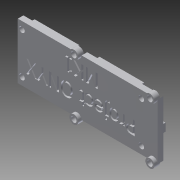
# Autodesk Inventor part: RearCarriageCarrierPlate
Saved by Autodesk Inventor 2015 (Build 190159000, 159)
## iProperties
Created: 2015-05-13
Part Number: RearCarriageCarrierPlate
Material: ABS Plastic
Document SubType Name: Modeling
Designer: Quinn
Density: 1.06 g/cm^3
Appearance: Smooth - White
Author: Quinn
Autodesk Inventor part; units mm, degrees
ref_plane "YZ Plane" through (0, 0, 0) normal (1, 0, 0) x (0, 1, 0)
ref_plane "XZ Plane" through (0, 0, 0) normal (0, 1, 0) x (-1, 0, 0)
ref_plane "XY Plane" through (0, 0, 0) normal (0, 0, 1) x (1, 0, 0)
sketch "Sketch1" plane through (0, 0, 0) normal (0, 1, 0) x (-1, 0, 0)
  line L0 (57, 25) -> (-57, 25)
  line L1 (-57, 25) -> (-57, -25)
  line L2 (-57, -25) -> (57, -25)
  line L3 (57, -25) -> (57, 25)
  point P0 (0, 0)
  point P1 (0, -25)
  point P2 (-57, 0)
  dimension "d0" = 114
  dimension "d1" = 50
  constraints: 8 end point, 2 midpoint, 2 parallel, 1 horizontal, 1 horizontal alignment, 1 perpendicular, 1 vertical alignment
  measures "d0" distance of L2.end L1.end
  measures "d1" distance of L1.end L0.end
extrude "Extrusion1" add sketch "Sketch1" along normal blind 5
sketch "Sketch2" plane through (0, 5, 0) normal (0, 1, 0) x (1, 0, 0)
  line L0 (-57, -25) -> (57, -25) projected
  line L1 (57, -25) -> (57, 25) projected
  line L2 (57, 25) -> (-57, 25) projected
  line L3 (-57, 25) -> (-57, -25) projected
  line L4 (57, -25) -> (49, -25)
  line L5 (49, -25) -> (49, 25)
  line L6 (49, 25) -> (57, 25)
  line L7 (57, 25) -> (57, -25)
  line L8 (49, -25) -> (9, -25)
  line L9 (9, -25) -> (9, 25)
  line L10 (9, 25) -> (49, 25)
  line L11 (49, 25) -> (49, -25)
  line L12 (-57, -25) -> (-49, -25)
  line L13 (-49, -25) -> (-49, 25)
  line L14 (-49, 25) -> (-57, 25)
  line L15 (-57, 25) -> (-57, -25)
  line L16 (-49, -25) -> (-9, -25)
  line L17 (-9, -25) -> (-9, 25)
  line L18 (-9, 25) -> (-49, 25)
  line L19 (-49, 25) -> (-49, -25)
  point P0 (0, 0)
  dimension "d4" = 8
  dimension "d5" = 40
  dimension "d6" = 8
  dimension "d7" = 40
  constraints: 32 end point, 8 parallel, 4 horizontal, 4 perpendicular, 4 point on line
  measures "d4" distance of L5.end L6.end
  measures "d5" distance of L9.end L10.end
  measures "d6" distance of L14.end L13.end
  measures "d7" distance of L18.end L17.end
extrude "Extrusion2" add sketch "Sketch2" along normal blind 2 contours L13 L2 L17 L0 | L9 L2 L5 L0
sketch "Sketch3" plane through (0, 0, 0) normal (0, -1, 0) x (1, 0, 0)
  line L0 (-57, 25) -> (57, 25) projected
  line L1 (-57, -25) -> (-57, 25) projected
  line L2 (57, -25) -> (-57, -25) projected
  line L3 (57, 25) -> (57, -25) projected
  line L4 (-57, 0) -> (57, 0)
  line L5 (-57, -25) -> (-57, -12.5)
  point P0 (0, 0)
  constraints: 4 end point, 2 midpoint, 1 point on line
sketch "Sketch4" plane through (0, 5, 0) normal (0, 1, 0) x (1, 0, 0)
  line L0 (9, -25) -> (9, 25) projected
  line L1 (9, 25) -> (-9, 25) projected
  line L2 (-9, 25) -> (-9, -25) projected
  line L3 (-9, -25) -> (9, -25) projected
  line L4 (49, 25) -> (49, -25) projected
  line L5 (49, -25) -> (57, -25) projected
  line L6 (57, -25) -> (57, 25) projected
  line L7 (57, 25) -> (49, 25) projected
  line L8 (-49, -25) -> (-49, 25) projected
  line L9 (-49, 25) -> (-57, 25) projected
  line L10 (-57, 25) -> (-57, -25) projected
  line L11 (-57, -25) -> (-49, -25) projected
  line L12 (-57, 3.5) -> (-49, 3.5)
  line L13 (-49, 3.5) -> (-49, -3.5)
  line L14 (-49, -3.5) -> (-57, -3.5)
  line L15 (-57, -3.5) -> (-57, 3.5)
  line L16 (-57, 3.5) -> (-49, -3.5) construction
  line L17 (-49, 3.5) -> (-57, -3.5) construction
  line L18 (-9, 3.5) -> (9, 3.5)
  line L19 (9, 3.5) -> (9, -3.5)
  line L20 (9, -3.5) -> (-9, -3.5)
  line L21 (-9, -3.5) -> (-9, 3.5)
  line L22 (-9, 3.5) -> (9, -3.5) construction
  line L23 (9, 3.5) -> (-9, -3.5) construction
  line L24 (49, 3.5) -> (57, 3.5)
  line L25 (57, 3.5) -> (57, -3.5)
  line L26 (57, -3.5) -> (49, -3.5)
  line L27 (49, -3.5) -> (49, 3.5)
  line L28 (49, 3.5) -> (57, -3.5) construction
  line L29 (57, 3.5) -> (49, -3.5) construction
  point P0 (0, 0)
  point P1 (-53, 0)
  point P2 (53, 0)
  dimension "d11" = 7
  constraints: 36 end point, 6 midpoint, 6 parallel, 5 point on line, 3 horizontal, 3 perpendicular
  measures "d11" distance of L12.end L13.end
extrude "Extrusion3" add sketch "Sketch4" along normal blind 2 contours L20 L2 L18 L0 | L24 L6 L26 L4 | L14 L10 L12 L8
sketch "Sketch5" plane through (0, 0, 0) normal (0, -1, 0) x (1, 0, 0)
  line L0 (-57, 25) -> (57, 25) projected
  line L1 (-57, -25) -> (-57, 25) projected
  line L2 (57, -25) -> (-57, -25) projected
  line L3 (57, 25) -> (57, -25) projected
  line L4 (-9, -25) -> (-49, -25) projected
  line L5 (-49, -25) -> (-49, -3.5) projected
  line L6 (-49, -3.5) -> (-57, -3.5) projected
  line L7 (-57, -3.5) -> (-57, 3.5) projected
  line L8 (-57, 3.5) -> (-49, 3.5) projected
  line L9 (-49, 3.5) -> (-49, 25) projected
  line L10 (-49, 25) -> (-9, 25) projected
  line L11 (-9, 25) -> (-9, 3.5) projected
  line L12 (-9, 3.5) -> (9, 3.5) projected
  line L13 (9, 3.5) -> (9, 25) projected
  line L14 (9, 25) -> (49, 25) projected
  line L15 (49, 25) -> (49, 3.5) projected
  line L16 (49, 3.5) -> (57, 3.5) projected
  line L17 (57, 3.5) -> (57, -3.5) projected
  line L18 (57, -3.5) -> (49, -3.5) projected
  line L19 (49, -3.5) -> (49, -25) projected
  line L20 (49, -25) -> (9, -25) projected
  line L21 (9, -25) -> (9, -3.5) projected
  line L22 (9, -3.5) -> (-9, -3.5) projected
  line L23 (-9, -3.5) -> (-9, -25) projected
  line L24 (-9, 25) -> (-4, 25)
  line L25 (-4, 25) -> (-4, -25)
  circle A0 centre (-4, -25) radius 4
  circle A1 centre (-4, 25) radius 4
  circle A2 centre (-4, 25) radius 2.5
  circle A3 centre (-4, -25) radius 2.5
  line L26 (-4, -25) -> (64, -25)
  line L27 (64, -25) -> (64, 25)
  circle A4 centre (64, -25) radius 4
  circle A5 centre (64, 25) radius 4
  circle A6 centre (64, -25) radius 2.5
  circle A7 centre (64, 25) radius 2.5
  point P0 (0, 0)
  dimension "d14" = 5
  dimension "d15" = 8
  dimension "d16" = 8
  dimension "d17" = 5
  dimension "d18" = 5
  dimension "d19" = 68
  dimension "d20" = 8
  dimension "d21" = 8
  dimension "d22" = 5
  dimension "d23" = 5
  constraints: 8 centre point, 8 coincident, 8 end point, 3 point on line, 2 perpendicular
  measures "d14" distance of L10.end L24.end
  measures "d15" diameter of A0
  measures "d16" diameter of A1
  measures "d17" diameter of A2
  measures "d18" diameter of A3
  measures "d19" distance of L26.start L26.end
  measures "d20" diameter of A4
  measures "d21" diameter of A5
  measures "d22" diameter of A6
  measures "d23" diameter of A7
move faces "Move1" translate (11, 0, 0) faces at (57, 1.6667, 1.1667)
extrude "Extrusion4" cut sketch "Sketch5" against normal blind 5 contours A2 L0 | L0 L25 A2 | L0 A2 L25 | A3 L2 L25 | L25 L2 A3 | L2 A3 | A6 L27 L26 | L26 L27 A6 | A7
extrude "Extrusion5" add sketch "Sketch5" against normal blind 5 contours A1 L0 A2 | L0 A2 L25 A1 | A1 L25 A2 L0 | A0 L2 A3 L25 | L25 A3 L2 A0 | L2 A3 A0 | A4 L27 A6 L26 | L26 A6 L27 A4 | A5
extrude "Extrusion6" add sketch "Sketch5" along normal blind 3 contours A1 L0 A2 | L0 A2 L25 A1 | A1 L25 A2 L0 | A0 L2 A3 L25 | L25 A3 L2 A0 | L2 A3 A0 | A4 L27 A6 L26 | L26 A6 L27 A4 | A5
sketch "Sketch6" plane through (0, 0, 0) normal (0, -1, 0) x (1, 0, 0)
  arc A0 (-8, 25) -> (0, 25) centre (-4, 25) ccw projected
  line L0 (-57, 25) -> (-8, 25) projected
  line L1 (-57, -25) -> (-57, 25) projected
  line L2 (-8, -25) -> (-57, -25) projected
  arc A1 (0, -25) -> (-8, -25) centre (-4, -25) ccw projected
  line L3 (60, -25) -> (0, -25) projected
  arc A2 (68, -25) -> (60, -25) centre (64, -25) ccw projected
  line L4 (68, 25) -> (68, -25) projected
  arc A3 (60, 25) -> (68, 25) centre (64, 25) ccw projected
  line L5 (0, 25) -> (60, 25) projected
  line L6 (185.6734, -14.1018) -> (-186.4568, -14.1018) construction
  line L7 (-186.4568, -14.1018) -> (-186.4568, 105.3716) construction
  line L8 (-186.4568, 105.3716) -> (185.6734, 105.3716) construction
  line L9 (185.6734, 105.3716) -> (185.6734, -14.1018) construction
  spline S0 degree 2 poles (39.8019, -10.2039) (39.8019, -9.4204) (40.3601, -8.0101) (40.8596, -7.5204) knots 0 0 0 1 2 2 2
  spline S1 degree 2 poles (40.8596, -7.5204) (41.4864, -6.9034) (43.1807, -6.2668) (44.4735, -6.2668) knots 0 0 0 1 2 2 2
  line L10 (44.4735, -6.2668) -> (45.8348, -6.2668)
  line L11 (45.8348, -6.2668) -> (45.8348, -1.7616)
  line L12 (45.8348, -1.7616) -> (47.441, -1.7616)
  line L13 (47.441, -1.7616) -> (47.441, -13.8471)
  line L14 (47.441, -13.8471) -> (44.4049, -13.8471)
  spline S2 degree 2 poles (44.4049, -13.8471) (43.3276, -13.8471) (41.8194, -13.4946) (41.2416, -13.093) knots 0 0 0 1 2 2 2
  spline S3 degree 2 poles (41.2416, -13.093) (40.5658, -12.6327) (39.8019, -11.2126) (39.8019, -10.2039) knots 0 0 0 1 2 2 2
  spline S4 degree 2 poles (41.4766, -10.1549) (41.4766, -10.7817) (41.9075, -11.7023) (42.3483, -11.9961) knots 0 0 0 1 2 2 2
  spline S5 degree 2 poles (42.3483, -11.9961) (42.7302, -12.2508) (43.7488, -12.4564) (44.5029, -12.4564) knots 0 0 0 1 2 2 2
  line L15 (44.5029, -12.4564) -> (45.8348, -12.4564)
  line L16 (45.8348, -12.4564) -> (45.8348, -7.6379)
  line L17 (45.8348, -7.6379) -> (44.7379, -7.6379)
  spline S6 degree 2 poles (44.7379, -7.6379) (43.7586, -7.6379) (42.5539, -7.9513) (42.1622, -8.3626) knots 0 0 0 1 2 2 2
  spline S7 degree 2 poles (42.1622, -8.3626) (41.7998, -8.725) (41.4766, -9.5771) (41.4766, -10.1549) knots 0 0 0 1 2 2 2
  line L18 (33.5828, -9.1951) -> (33.6612, -9.1951)
  spline S8 degree 2 poles (33.6612, -9.1951) (33.8375, -9.2441) (34.2194, -9.2637) (34.4839, -9.2637) knots 0 0 0 1 2 2 2
  spline S9 degree 2 poles (34.4839, -9.2637) (35.1009, -9.2637) (36.3153, -8.725) (36.8637, -8.1961) knots 0 0 0 1 2 2 2
  line L19 (36.8637, -8.1961) -> (36.8637, -1.7616)
  line L20 (36.8637, -1.7616) -> (38.3916, -1.7616)
  line L21 (38.3916, -1.7616) -> (38.3916, -10.8307)
  line L22 (38.3916, -10.8307) -> (36.8637, -10.8307)
  line L23 (36.8637, -10.8307) -> (36.8637, -9.4791)
  spline S10 degree 2 poles (36.8637, -9.4791) (36.0313, -10.2234) (34.7875, -10.8307) (34.1998, -10.8307) knots 0 0 0 1 2 2 2
  spline S11 degree 2 poles (34.1998, -10.8307) (33.9648, -10.8307) (33.7297, -10.8111) (33.5828, -10.7817) knots 0 0 0 1 2 2 2
  line L24 (33.5828, -10.7817) -> (33.5828, -9.1951)
  spline S12 degree 2 poles (24.9447, -6.2961) (24.9447, -4.0044) (27.1483, -1.507) (28.9896, -1.507) knots 0 0 0 1 2 2 2
  spline S13 degree 2 poles (28.9896, -1.507) (30.8798, -1.507) (33.0442, -4.0828) (33.0442, -6.2961) knots 0 0 0 1 2 2 2
  spline S14 degree 2 poles (33.0442, -6.2961) (33.0442, -8.5683) (30.8112, -11.0853) (28.9896, -11.0853) knots 0 0 0 1 2 2 2
  spline S15 degree 2 poles (28.9896, -11.0853) (27.1483, -11.0853) (24.9447, -8.5781) (24.9447, -6.2961) knots 0 0 0 1 2 2 2
  spline S16 degree 2 poles (26.5215, -6.2961) (26.5215, -8.059) (27.8045, -9.7729) (28.9896, -9.7729) knots 0 0 0 1 2 2 2
  spline S17 degree 2 poles (28.9896, -9.7729) (30.1746, -9.7729) (31.4674, -8.059) (31.4674, -6.2961) knots 0 0 0 1 2 2 2
  spline S18 degree 2 poles (31.4674, -6.2961) (31.4674, -4.5822) (30.1746, -2.8194) (28.9896, -2.8194) knots 0 0 0 1 2 2 2
  spline S19 degree 2 poles (28.9896, -2.8194) (27.8143, -2.8194) (26.5215, -4.5529) (26.5215, -6.2961) knots 0 0 0 1 2 2 2
  spline S20 degree 2 poles (20.9097, -1.507) (20.9097, 0.0404) (22.5747, 1.6662) (24.0339, 1.6662) knots 0 0 0 1 2 2 2
  spline S21 degree 2 poles (24.0339, 1.6662) (24.2886, 1.6662) (24.9154, 1.6172) (25.219, 1.5682) knots 0 0 0 1 2 2 2
  line L25 (25.219, 1.5682) -> (25.219, 0.1971)
  line L26 (25.219, 0.1971) -> (25.1308, 0.1971)
  spline S22 degree 2 poles (25.1308, 0.1971) (24.9545, 0.2363) (24.5236, 0.3146) (24.3277, 0.3146) knots 0 0 0 1 2 2 2
  spline S23 degree 2 poles (24.3277, 0.3146) (23.7205, 0.3146) (22.9272, 0.011) (22.7411, -0.3122) knots 0 0 0 1 2 2 2
  spline S24 degree 2 poles (22.7411, -0.3122) (22.5551, -0.606) (22.4375, -1.4972) (22.4375, -2.1338) knots 0 0 0 1 2 2 2
  line L27 (22.4375, -2.1338) -> (22.4375, -9.5673)
  line L28 (22.4375, -9.5673) -> (24.0731, -9.5673)
  line L29 (24.0731, -9.5673) -> (24.0731, -10.8307)
  line L30 (24.0731, -10.8307) -> (20.9097, -10.8307)
  line L31 (20.9097, -10.8307) -> (20.9097, -1.507)
  line L32 (20.8999, -12.3389) -> (22.6334, -12.3389)
  line L33 (22.6334, -12.3389) -> (22.6334, -13.9255)
  line L34 (22.6334, -13.9255) -> (20.8999, -13.9255)
  line L35 (20.8999, -13.9255) -> (20.8999, -12.3389)
  spline S25 degree 2 poles (14.7592, -1.556) (16.9334, -1.556) (19.3231, -3.9946) (19.3231, -6.2472) knots 0 0 0 1 2 2 2
  spline S26 degree 2 poles (19.3231, -6.2472) (19.3231, -8.4606) (17.002, -11.0853) (15.1314, -11.0853) knots 0 0 0 1 2 2 2
  spline S27 degree 2 poles (15.1314, -11.0853) (14.2891, -11.0853) (12.9866, -10.5956) (12.5067, -10.0765) knots 0 0 0 1 2 2 2
  spline S28 degree 2 poles (12.5067, -10.0765) (12.017, -9.5575) (11.4979, -8.059) (11.4979, -6.9719) knots 0 0 0 1 2 2 2
  line L36 (11.4979, -6.9719) -> (11.4979, -6.1394)
  line L37 (11.4979, -6.1394) -> (17.7757, -6.1394)
  spline S29 degree 2 poles (17.7757, -6.1394) (17.7757, -4.5627) (16.1891, -2.8879) (14.7788, -2.8879) knots 0 0 0 1 2 2 2
  spline S30 degree 2 poles (14.7788, -2.8879) (14.2793, -2.8879) (13.3098, -3.1132) (12.918, -3.2895) knots 0 0 0 1 2 2 2
  spline S31 degree 2 poles (12.918, -3.2895) (12.5067, -3.4853) (11.9386, -3.8281) (11.7525, -3.9848) knots 0 0 0 1 2 2 2
  line L38 (11.7525, -3.9848) -> (11.6644, -3.9848)
  line L39 (11.6644, -3.9848) -> (11.6644, -2.3199)
  spline S32 degree 2 poles (11.6644, -2.3199) (11.9288, -2.2122) (12.7319, -1.8988) (13.0453, -1.8106) knots 0 0 0 1 2 2 2
  spline S33 degree 2 poles (13.0453, -1.8106) (13.486, -1.6833) (14.2108, -1.556) (14.7592, -1.556) knots 0 0 0 1 2 2 2
  spline S34 degree 2 poles (12.9866, -7.3049) (13.0061, -7.9219) (13.2608, -8.8229) (13.5056, -9.1265) knots 0 0 0 1 2 2 2
  spline S35 degree 2 poles (13.5056, -9.1265) (13.7701, -9.4693) (14.6025, -9.8317) (15.2195, -9.8317) knots 0 0 0 1 2 2 2
  spline S36 degree 2 poles (15.2195, -9.8317) (15.8268, -9.8317) (16.6788, -9.4693) (17.0314, -9.1168) knots 0 0 0 1 2 2 2
  spline S37 degree 2 poles (17.0314, -9.1168) (17.3742, -8.7544) (17.7267, -7.8827) (17.7757, -7.3049) knots 0 0 0 1 2 2 2
  line L40 (17.7757, -7.3049) -> (12.9866, -7.3049)
  spline S38 degree 2 poles (6.3464, -1.556) (7.2866, -1.556) (8.8438, -2.1338) (9.402, -2.7214) knots 0 0 0 1 2 2 2
  spline S39 degree 2 poles (9.402, -2.7214) (9.9603, -3.2993) (10.5773, -5.0817) (10.5773, -6.2766) knots 0 0 0 1 2 2 2
  spline S40 degree 2 poles (10.5773, -6.2766) (10.5773, -7.4714) (9.9407, -9.2147) (9.402, -9.8023) knots 0 0 0 1 2 2 2
  spline S41 degree 2 poles (9.402, -9.8023) (8.8634, -10.3997) (7.267, -11.0363) (6.3464, -11.0363) knots 0 0 0 1 2 2 2
  spline S42 degree 2 poles (6.3464, -11.0363) (5.6021, -11.0363) (4.2114, -10.6152) (3.6727, -10.341) knots 0 0 0 1 2 2 2
  line L41 (3.6727, -10.341) -> (3.6727, -8.6271)
  line L42 (3.6727, -8.6271) -> (3.7608, -8.6271)
  spline S43 degree 2 poles (3.7608, -8.6271) (3.9273, -8.7642) (4.4366, -9.1168) (4.799, -9.3028) knots 0 0 0 1 2 2 2
  spline S44 degree 2 poles (4.799, -9.3028) (5.1222, -9.4595) (5.984, -9.7044) (6.3758, -9.7044) knots 0 0 0 1 2 2 2
  spline S45 degree 2 poles (6.3758, -9.7044) (7.5608, -9.7044) (9.0005, -7.9121) (9.0005, -6.2766) knots 0 0 0 1 2 2 2
  spline S46 degree 2 poles (9.0005, -6.2766) (9.0005, -4.6802) (7.6098, -2.8879) (6.3758, -2.8879) knots 0 0 0 1 2 2 2
  spline S47 degree 2 poles (6.3758, -2.8879) (5.6314, -2.8879) (4.2799, -3.5049) (3.7608, -3.9848) knots 0 0 0 1 2 2 2
  line L43 (3.7608, -3.9848) -> (3.6727, -3.9848)
  line L44 (3.6727, -3.9848) -> (3.6727, -2.2709)
  spline S48 degree 2 poles (3.6727, -2.2709) (3.898, -2.1632) (4.5835, -1.8596) (4.8577, -1.791) knots 0 0 0 1 2 2 2
  spline S49 degree 2 poles (4.8577, -1.791) (5.2495, -1.6735) (5.8665, -1.556) (6.3464, -1.556) knots 0 0 0 1 2 2 2
  spline S50 degree 2 poles (-0.4603, -1.5854) (0.7835, -1.5854) (2.184, -3.0054) (2.184, -4.5431) knots 0 0 0 1 2 2 2
  line L45 (2.184, -4.5431) -> (2.184, -9.5673)
  line L46 (2.184, -9.5673) -> (3.2124, -9.5673)
  line L47 (3.2124, -9.5673) -> (3.2124, -10.8307)
  line L48 (3.2124, -10.8307) -> (2.184, -10.8307)
  line L49 (2.184, -10.8307) -> (2.184, -13.4358)
  line L50 (2.184, -13.4358) -> (0.6562, -13.4358)
  line L51 (0.6562, -13.4358) -> (0.6562, -10.8307)
  line L52 (0.6562, -10.8307) -> (-2.1546, -10.8307)
  line L53 (-2.1546, -10.8307) -> (-2.1546, -9.5673)
  line L54 (-2.1546, -9.5673) -> (0.6562, -9.5673)
  line L55 (0.6562, -9.5673) -> (0.6562, -5.2482)
  spline S51 degree 2 poles (0.6562, -5.2482) (0.6562, -4.5627) (0.6072, -3.8085) (0.4408, -3.4853) knots 0 0 0 1 2 2 2
  spline S52 degree 2 poles (0.4408, -3.4853) (0.3036, -3.2013) (-0.3134, -2.9173) (-0.8422, -2.9173) knots 0 0 0 1 2 2 2
  spline S53 degree 2 poles (-0.8422, -2.9173) (-1.2144, -2.9173) (-1.9097, -3.1426) (-2.0664, -3.2111) knots 0 0 0 1 2 2 2
  line L56 (-2.0664, -3.2111) -> (-2.1546, -3.2111)
  line L57 (-2.1546, -3.2111) -> (-2.1546, -1.84)
  spline S54 degree 2 poles (-2.1546, -1.84) (-1.7237, -1.7225) (-0.8422, -1.5854) (-0.4603, -1.5854) knots 0 0 0 1 2 2 2
  spline S55 degree 2 poles (-17.139, -12.4662) (-17.8246, -11.6631) (-18.5885, -9.3126) (-18.5885, -7.8044) knots 0 0 0 1 2 2 2
  spline S56 degree 2 poles (-18.5885, -7.8044) (-18.5885, -6.3353) (-17.8442, -3.9554) (-17.139, -3.1524) knots 0 0 0 1 2 2 2
  spline S57 degree 2 poles (-17.139, -3.1524) (-16.3947, -2.3101) (-14.4262, -1.507) (-13.2411, -1.507) knots 0 0 0 1 2 2 2
  spline S58 degree 2 poles (-13.2411, -1.507) (-12.0169, -1.507) (-10.0582, -2.3395) (-9.3432, -3.1524) knots 0 0 0 1 2 2 2
  spline S59 degree 2 poles (-9.3432, -3.1524) (-8.6479, -3.9554) (-7.9035, -6.3157) (-7.9035, -7.8044) knots 0 0 0 1 2 2 2
  spline S60 degree 2 poles (-7.9035, -7.8044) (-7.9035, -9.3224) (-8.6576, -11.6337) (-9.353, -12.4662) knots 0 0 0 1 2 2 2
  spline S61 degree 2 poles (-9.353, -12.4662) (-10.0582, -13.2693) (-12.0267, -14.1018) (-13.2411, -14.1018) knots 0 0 0 1 2 2 2
  spline S62 degree 2 poles (-13.2411, -14.1018) (-14.4751, -14.1018) (-16.4535, -13.2399) (-17.139, -12.4662) knots 0 0 0 1 2 2 2
  spline S63 degree 2 poles (-16.9138, -7.8044) (-16.9138, -8.9992) (-16.3947, -10.8502) (-15.9246, -11.4575) knots 0 0 0 1 2 2 2
  spline S64 degree 2 poles (-15.9246, -11.4575) (-15.4447, -12.0843) (-14.0932, -12.7111) (-13.2509, -12.7111) knots 0 0 0 1 2 2 2
  spline S65 degree 2 poles (-13.2509, -12.7111) (-12.3793, -12.7111) (-11.0669, -12.1038) (-10.5674, -11.4575) knots 0 0 0 1 2 2 2
  spline S66 degree 2 poles (-10.5674, -11.4575) (-10.0875, -10.8405) (-9.5783, -8.9796) (-9.5783, -7.8044) knots 0 0 0 1 2 2 2
  spline S67 degree 2 poles (-9.5783, -7.8044) (-9.5783, -5.4245) (-11.5762, -2.8977) (-13.2509, -2.8977) knots 0 0 0 1 2 2 2
  spline S68 degree 2 poles (-13.2509, -2.8977) (-14.9257, -2.8977) (-16.9138, -5.4245) (-16.9138, -7.8044) knots 0 0 0 1 2 2 2
  line L58 (-28.9993, -1.7616) -> (-27.1972, -1.7616)
  line L59 (-27.1972, -1.7616) -> (-21.8498, -12.1822)
  line L60 (-21.8498, -12.1822) -> (-21.8498, -1.7616)
  line L61 (-21.8498, -1.7616) -> (-20.3514, -1.7616)
  line L62 (-20.3514, -1.7616) -> (-20.3514, -13.8471)
  line L63 (-20.3514, -13.8471) -> (-22.6333, -13.8471)
  line L64 (-22.6333, -13.8471) -> (-27.5008, -4.2786)
  line L65 (-27.5008, -4.2786) -> (-27.5008, -13.8471)
  line L66 (-27.5008, -13.8471) -> (-28.9993, -13.8471)
  line L67 (-28.9993, -13.8471) -> (-28.9993, -1.7616)
  line L68 (-39.9095, -13.8471) -> (-35.8255, -7.109)
  line L69 (-35.8255, -7.109) -> (-35.8255, -1.7616)
  line L70 (-35.8255, -1.7616) -> (-34.2194, -1.7616)
  line L71 (-34.2194, -1.7616) -> (-34.2194, -6.9425)
  line L72 (-34.2194, -6.9425) -> (-30.1354, -13.8471)
  line L73 (-30.1354, -13.8471) -> (-31.9178, -13.8471)
  line L74 (-31.9178, -13.8471) -> (-35.0322, -8.5291)
  line L75 (-35.0322, -8.5291) -> (-38.2054, -13.8471)
  line L76 (-38.2054, -13.8471) -> (-39.9095, -13.8471)
  line L77 (-49.3801, -1.7616) -> (-47.5389, -1.7616)
  line L78 (-47.5389, -1.7616) -> (-44.6007, -6.5802)
  line L79 (-44.6007, -6.5802) -> (-41.6039, -1.7616)
  line L80 (-41.6039, -1.7616) -> (-39.8704, -1.7616)
  line L81 (-39.8704, -1.7616) -> (-43.7193, -7.8142)
  line L82 (-43.7193, -7.8142) -> (-39.9879, -13.8471)
  line L83 (-39.9879, -13.8471) -> (-41.8291, -13.8471)
  line L84 (-41.8291, -13.8471) -> (-44.7085, -9.1168)
  line L85 (-44.7085, -9.1168) -> (-47.6466, -13.8471)
  line L86 (-47.6466, -13.8471) -> (-49.3801, -13.8471)
  line L87 (-49.3801, -13.8471) -> (-45.5997, -7.8925)
  line L88 (-45.5997, -7.8925) -> (-49.3801, -1.7616)
  line L89 (3.849, 18.1368) -> (5.4552, 18.1368)
  line L90 (5.4552, 18.1368) -> (5.4552, 7.7261)
  line L91 (5.4552, 7.7261) -> (8.6087, 14.8069)
  line L92 (8.6087, 14.8069) -> (9.5881, 14.8069)
  line L93 (9.5881, 14.8069) -> (12.7123, 7.7261)
  line L94 (12.7123, 7.7261) -> (12.7123, 18.1368)
  line L95 (12.7123, 18.1368) -> (14.2108, 18.1368)
  line L96 (14.2108, 18.1368) -> (14.2108, 6.0513)
  line L97 (14.2108, 6.0513) -> (12.017, 6.0513)
  line L98 (12.017, 6.0513) -> (9.0005, 12.7796)
  line L99 (9.0005, 12.7796) -> (6.082, 6.0513)
  line L100 (6.082, 6.0513) -> (3.849, 6.0513)
  line L101 (3.849, 6.0513) -> (3.849, 18.1368)
  line L102 (-7.4138, 18.1368) -> (-5.3278, 18.1368)
  line L103 (-5.3278, 18.1368) -> (-0.9108, 12.5152)
  line L104 (-0.9108, 12.5152) -> (-0.2056, 13.3085)
  line L105 (-0.2056, 13.3085) -> (-0.2056, 18.1368)
  line L106 (-0.2056, 18.1368) -> (1.4005, 18.1368)
  line L107 (1.4005, 18.1368) -> (1.4005, 6.0513)
  line L108 (1.4005, 6.0513) -> (-0.2056, 6.0513)
  line L109 (-0.2056, 6.0513) -> (-0.2056, 11.6044)
  line L110 (-0.2056, 11.6044) -> (-5.1613, 6.0513)
  line L111 (-5.1613, 6.0513) -> (-7.12, 6.0513)
  line L112 (-7.12, 6.0513) -> (-2.1154, 11.4477)
  line L113 (-2.1154, 11.4477) -> (-7.4138, 18.1368)
  line L114 (-14.8767, 18.1368) -> (-8.9808, 18.1368)
  line L115 (-8.9808, 18.1368) -> (-8.9808, 16.9028)
  line L116 (-8.9808, 16.9028) -> (-11.1746, 16.9028)
  line L117 (-11.1746, 16.9028) -> (-11.1746, 8.8034)
  line L118 (-11.1746, 8.8034) -> (-8.9808, 8.8034)
  line L119 (-8.9808, 8.8034) -> (-8.9808, 7.6967)
  spline S69 degree 2 poles (-8.9808, 7.6967) (-10.2247, 7.6967) (-11.3999, 6.9915) (-11.4783, 6.0121) knots 0 0 0 1 2 2 2
  line L120 (-11.4783, 6.0121) -> (-12.7319, 6.0121)
  line L121 (-12.7319, 6.0121) -> (-12.7319, 16.9028)
  line L122 (-12.7319, 16.9028) -> (-14.8767, 16.9028)
  line L123 (-14.8767, 16.9028) -> (-14.8767, 18.1368)
  point P0 (0, 0)
  constraints: 2 other
emboss "Emboss1" sketch "Sketch6" operation cut depth 2 direction (0, 1, 0) contours S0 S1 L10 L11 L12 L13 L14 S2 S3 | L18 S8 S9 L19 L20 L21 L22 L23 S10 S11 L24 | S12 S13 S14 S15 | S20 S21 L25 L26 S22 S23 S24 L27 L28 L29 L30 L31 | L32 L33 L34 L35 | S25 S26 S27 S28 L36 L37 S29 S30 S31 L38 L39 S32 S33 | S38 S39 S40 S41 S42 L41 L42 S43 S44 S45 S46 S47 L43 L44 S48 S49 | S50 L45 L46 L47 L48 L49 L50 L51 L52 L53 L54 L55 S51 S52 S53 L56 L57 S54 | S55 S56 S57 S58 S59 S60 S61 S62 | L58 L59 L60 L61 L62 L63 L64 L65 L66 L67 | L68 L69 L70 L71 L72 L73 L74 L75 L76 | L77 L78 L79 L80 L81 L82 L83 L84 L85 L86 L87 L88 | L89 L90 L91 L92 L93 L94 L95 L96 L97 L98 L99 L100 L101 | L102 L103 L104 L105 L106 L107 L108 L109 L110 L111 L112 L113 | L114 L115 L116 L117 L118 L119 S69 L120 L121 L122 L123
sketch "Sketch7" plane through (0, 0, 0) normal (0, -1, 0) x (1, 0, 0)
  line L0 (-11.4783, 6.0121) -> (-12.7319, 6.0121) projected
  line L1 (-12.7319, 6.0121) -> (-12.7319, 16.9028) projected
  line L2 (-12.7319, 16.9028) -> (-14.8767, 16.9028) projected
  line L3 (-14.8767, 16.9028) -> (-14.8767, 18.1368) projected
  line L4 (-14.8767, 18.1368) -> (-8.9808, 18.1368) projected
  line L5 (-8.9808, 18.1368) -> (-8.9808, 16.9028) projected
  line L6 (-8.9808, 16.9028) -> (-11.1746, 16.9028) projected
  line L7 (-11.1746, 16.9028) -> (-11.1746, 8.8034) projected
  line L8 (-11.1746, 8.8034) -> (-8.9808, 8.8034) projected
  line L9 (-8.9808, 8.8034) -> (-8.9808, 7.6967) projected
  line L10 (22.4375, -2.1338) -> (22.4375, -9.5673) projected
  line L11 (22.4375, -9.5673) -> (24.0731, -9.5673) projected
  line L12 (24.0731, -9.5673) -> (24.0731, -10.8307) projected
  line L13 (24.0731, -10.8307) -> (20.9097, -10.8307) projected
  line L14 (20.9097, -10.8307) -> (20.9097, -1.507) projected
  line L15 (25.219, 1.5682) -> (25.219, 0.1971) projected
  line L16 (25.219, 0.1971) -> (25.1308, 0.1971) projected
  line L17 (47.441, -13.8471) -> (44.4049, -13.8471) projected
  line L18 (44.4735, -6.2668) -> (45.8348, -6.2668) projected
  line L19 (45.8348, -6.2668) -> (45.8348, -1.7616) projected
  line L20 (45.8348, -1.7616) -> (47.441, -1.7616) projected
  line L21 (47.441, -1.7616) -> (47.441, -13.8471) projected
  line L22 (11.7525, -3.9848) -> (11.6644, -3.9848) projected
  line L23 (11.6644, -3.9848) -> (11.6644, -2.3199) projected
  line L24 (11.4979, -6.9719) -> (11.4979, -6.1394) projected
  line L25 (11.4979, -6.1394) -> (17.7757, -6.1394) projected
  line L26 (36.8637, -10.8307) -> (36.8637, -9.4791) projected
  line L27 (33.5828, -10.7817) -> (33.5828, -9.1951) projected
  line L28 (33.5828, -9.1951) -> (33.6612, -9.1951) projected
  line L29 (36.8637, -8.1961) -> (36.8637, -1.7616) projected
  line L30 (36.8637, -1.7616) -> (38.3916, -1.7616) projected
  line L31 (38.3916, -1.7616) -> (38.3916, -10.8307) projected
  line L32 (38.3916, -10.8307) -> (36.8637, -10.8307) projected
  line L33 (3.7608, -3.9848) -> (3.6727, -3.9848) projected
  line L34 (3.6727, -3.9848) -> (3.6727, -2.2709) projected
  line L35 (3.6727, -10.341) -> (3.6727, -8.6271) projected
  line L36 (3.6727, -8.6271) -> (3.7608, -8.6271) projected
  line L37 (20.8999, -12.3389) -> (22.6334, -12.3389) projected
  line L38 (22.6334, -12.3389) -> (22.6334, -13.9255) projected
  line L39 (22.6334, -13.9255) -> (20.8999, -13.9255) projected
  line L40 (20.8999, -13.9255) -> (20.8999, -12.3389) projected
  line L41 (0.6562, -9.5673) -> (0.6562, -5.2482) projected
  line L42 (-2.0664, -3.2111) -> (-2.1546, -3.2111) projected
  line L43 (-2.1546, -3.2111) -> (-2.1546, -1.84) projected
  line L44 (2.184, -4.5431) -> (2.184, -9.5673) projected
  line L45 (2.184, -9.5673) -> (3.2124, -9.5673) projected
  line L46 (3.2124, -9.5673) -> (3.2124, -10.8307) projected
  line L47 (3.2124, -10.8307) -> (2.184, -10.8307) projected
  line L48 (2.184, -10.8307) -> (2.184, -13.4358) projected
  line L49 (2.184, -13.4358) -> (0.6562, -13.4358) projected
  line L50 (0.6562, -13.4358) -> (0.6562, -10.8307) projected
  line L51 (0.6562, -10.8307) -> (-2.1546, -10.8307) projected
  line L52 (-2.1546, -10.8307) -> (-2.1546, -9.5673) projected
  line L53 (-2.1546, -9.5673) -> (0.6562, -9.5673) projected
  line L54 (-22.6333, -13.8471) -> (-27.5008, -4.2786) projected
  line L55 (-27.5008, -4.2786) -> (-27.5008, -13.8471) projected
  line L56 (-27.5008, -13.8471) -> (-28.9993, -13.8471) projected
  line L57 (-28.9993, -13.8471) -> (-28.9993, -1.7616) projected
  line L58 (-28.9993, -1.7616) -> (-27.1972, -1.7616) projected
  line L59 (-27.1972, -1.7616) -> (-21.8498, -12.1822) projected
  line L60 (-21.8498, -12.1822) -> (-21.8498, -1.7616) projected
  line L61 (-21.8498, -1.7616) -> (-20.3514, -1.7616) projected
  line L62 (-20.3514, -1.7616) -> (-20.3514, -13.8471) projected
  line L63 (-20.3514, -13.8471) -> (-22.6333, -13.8471) projected
  line L64 (-31.9178, -13.8471) -> (-35.0322, -8.5291) projected
  line L65 (-35.0322, -8.5291) -> (-38.2054, -13.8471) projected
  line L66 (-38.2054, -13.8471) -> (-39.9095, -13.8471) projected
  line L67 (-39.9095, -13.8471) -> (-35.8255, -7.109) projected
  line L68 (-35.8255, -7.109) -> (-35.8255, -1.7616) projected
  line L69 (-35.8255, -1.7616) -> (-34.2194, -1.7616) projected
  line L70 (-34.2194, -1.7616) -> (-34.2194, -6.9425) projected
  line L71 (-34.2194, -6.9425) -> (-30.1354, -13.8471) projected
  line L72 (-30.1354, -13.8471) -> (-31.9178, -13.8471) projected
  line L73 (-41.8291, -13.8471) -> (-44.7085, -9.1168) projected
  line L74 (-44.7085, -9.1168) -> (-47.6466, -13.8471) projected
  line L75 (-47.6466, -13.8471) -> (-49.3801, -13.8471) projected
  line L76 (-49.3801, -13.8471) -> (-45.5997, -7.8925) projected
  line L77 (-45.5997, -7.8925) -> (-49.3801, -1.7616) projected
  line L78 (-49.3801, -1.7616) -> (-47.5389, -1.7616) projected
  line L79 (-47.5389, -1.7616) -> (-44.6007, -6.5802) projected
  line L80 (-44.6007, -6.5802) -> (-41.6039, -1.7616) projected
  line L81 (-41.6039, -1.7616) -> (-39.8704, -1.7616) projected
  line L82 (-39.8704, -1.7616) -> (-43.7193, -7.8142) projected
  line L83 (-43.7193, -7.8142) -> (-39.9879, -13.8471) projected
  line L84 (-39.9879, -13.8471) -> (-41.8291, -13.8471) projected
  line L85 (14.2108, 6.0513) -> (12.017, 6.0513) projected
  line L86 (12.017, 6.0513) -> (9.0005, 12.7796) projected
  line L87 (9.0005, 12.7796) -> (6.082, 6.0513) projected
  line L88 (6.082, 6.0513) -> (3.849, 6.0513) projected
  line L89 (3.849, 6.0513) -> (3.849, 18.1368) projected
  line L90 (3.849, 18.1368) -> (5.4552, 18.1368) projected
  line L91 (5.4552, 18.1368) -> (5.4552, 7.7261) projected
  line L92 (5.4552, 7.7261) -> (8.6087, 14.8069) projected
  line L93 (8.6087, 14.8069) -> (9.5881, 14.8069) projected
  line L94 (9.5881, 14.8069) -> (12.7123, 7.7261) projected
  line L95 (12.7123, 7.7261) -> (12.7123, 18.1368) projected
  line L96 (12.7123, 18.1368) -> (14.2108, 18.1368) projected
  line L97 (14.2108, 18.1368) -> (14.2108, 6.0513) projected
  line L98 (-0.2056, 6.0513) -> (-0.2056, 11.6044) projected
  line L99 (-0.2056, 11.6044) -> (-5.1613, 6.0513) projected
  line L100 (-5.1613, 6.0513) -> (-7.12, 6.0513) projected
  line L101 (-7.12, 6.0513) -> (-2.1154, 11.4477) projected
  line L102 (-2.1154, 11.4477) -> (-7.4138, 18.1368) projected
  line L103 (-7.4138, 18.1368) -> (-5.3278, 18.1368) projected
  line L104 (-5.3278, 18.1368) -> (-0.9108, 12.5152) projected
  line L105 (-0.9108, 12.5152) -> (-0.2056, 13.3085) projected
  line L106 (-0.2056, 13.3085) -> (-0.2056, 18.1368) projected
  line L107 (-0.2056, 18.1368) -> (1.4005, 18.1368) projected
  line L108 (1.4005, 18.1368) -> (1.4005, 6.0513) projected
  line L109 (1.4005, 6.0513) -> (-0.2056, 6.0513) projected
  arc A0 (-8, 25) -> (0, 25) centre (-4, 25) ccw projected
  line L110 (-57, 25) -> (-8, 25) projected
  line L111 (-57, -25) -> (-57, 25) projected
  line L112 (-8, -25) -> (-57, -25) projected
  arc A1 (0, -25) -> (-8, -25) centre (-4, -25) ccw projected
  line L113 (60, -25) -> (0, -25) projected
  arc A2 (68, -25) -> (60, -25) centre (64, -25) ccw projected
  line L114 (68, 25) -> (68, -25) projected
  arc A3 (60, 25) -> (68, 25) centre (64, 25) ccw projected
  line L115 (0, 25) -> (60, 25) projected
  line L116 (-57, 0) -> (5.5, 0)
  line L117 (-53.318, -18.326) -> (53.318, -18.326)
  line L118 (53.318, -18.326) -> (53.318, 18.326)
  line L119 (53.318, 18.326) -> (-53.318, 18.326)
  line L120 (-53.318, 18.326) -> (-53.318, -18.326)
  line L121 (-53.318, -18.326) -> (53.318, 18.326) construction
  line L122 (53.318, -18.326) -> (-53.318, 18.326) construction
  circle A4 centre (-53.318, 18.326) radius 2.5
  circle A5 centre (-53.318, -18.326) radius 2.5
  circle A6 centre (53.318, -18.326) radius 2.5
  circle A7 centre (53.318, 18.326) radius 2.5
  point P0 (0, 0)
  dimension "d35" = 62.5
  dimension "d36" = 106.636
  dimension "d37" = 36.652
  dimension "d38" = 5
  dimension "d39" = 5
  dimension "d40" = 5
  dimension "d41" = 5
  constraints: 14 end point, 4 centre point, 4 coincident, 3 midpoint, 2 parallel, 2 perpendicular, 1 horizontal, 52 other
  measures "d35" distance of L116.start L116.end
  measures "d36" distance of L119.end L118.end
  measures "d37" distance of L118.end L117.end
  measures "d38" diameter of A4
  measures "d39" diameter of A5
  measures "d40" diameter of A6
  measures "d41" diameter of A7
extrude "Extrusion7" cut sketch "Sketch7" against normal through all contours L120 A5 L117 | L117 A5 L120 | A6 L118 L117 | L117 L118 A6 | A4 L119 L120 | L120 L119 A4 | A7 L119 L118 | L118 L119 A7
sketch "Sketch8" plane through (0, 5, 0) normal (0, 1, 0) x (1, 0, 0)
  circle A0 centre (64, -25) radius 4 projected
  circle A1 centre (-4, -25) radius 4 projected
  circle A2 centre (-4, 25) radius 4 projected
  circle A3 centre (64, 25) radius 4 projected
  point P0 (0, 0)
extrude "Extrusion8" cut sketch "Sketch8" against normal blind 3
body "Solid1"
